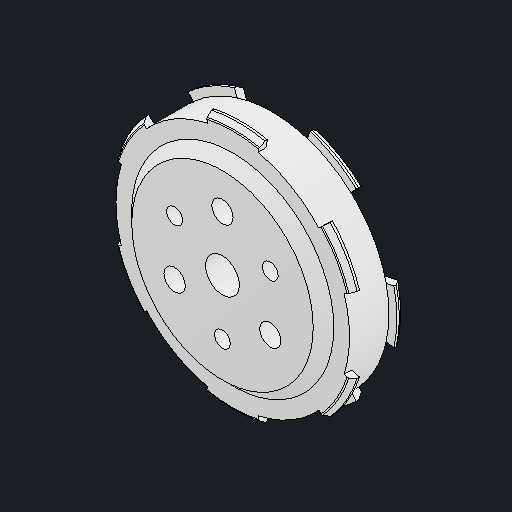
# Autodesk Inventor part: 36mm tamiya-slim-tire-wheel
Saved by Autodesk Inventor 2023.2 (Build 272271030, 271C)
## iProperties
Created: 2023-10-14
Part Number: 36mm tamiya-slim-tire-wheel
Material: Stainless Steel
Document SubType Name: Modeling
Designer: takag
Density: 8 g/cm^3
Appearance: 滑らか - 白
Author: takag
Autodesk Inventor part; units mm, degrees
ref_plane "YZ Plane" through (0, 0, 0) normal (1, 0, 0) x (0, 1, 0)
ref_plane "XZ Plane" through (0, 0, 0) normal (0, 1, 0) x (-1, 0, 0)
ref_plane "XY Plane" through (0, 0, 0) normal (0, 0, 1) x (1, 0, 0)
sketch "スケッチ1" plane through (0, 0, 0) normal (0, 0, 1) x (1, 0, 0)
  circle A0 centre (0, 0) radius 15.8
  dimension "d0" = 31.6
  constraints: 1 centre point, 1 coincident
  measures "d0" diameter of A0
extrude "押し出し1" add sketch "スケッチ1" along normal blind 7.3
sketch "スケッチ2" plane through (0, 0, 7.3) normal (0, 0, 1) x (1, 0, 0)
  circle A0 centre (0, 0) radius 12.8
  circle A1 centre (0, 0) radius 15.8 projected
  dimension "d3" = 3
  constraints: 1 centre point, 1 coincident
  measures "d3" radial gap between concentric circles of A1 A0
extrude "押し出し2" cut sketch "スケッチ2" against normal blind 1.3
sketch "スケッチ3" plane through (0, 0, 7.3) normal (0, 0, 1) x (1, 0, 0)
  circle A0 centre (0, 0) radius 13
  dimension "d6" = 26
  constraints: 1 centre point, 1 coincident
  measures "d6" diameter of A0
ref_plane "Work Plane2" through (0, 0, 7.3) normal (0, 0, 1) x (1, 0, 0)
sketch "スケッチ6" plane through (0, 0, 0) normal (1, 0, 0) x (0, 1, 0)
  line L0 (15.8, 0) -> (15.8, 6) projected
  line L1 (-15.8, 6) -> (15.8, 6) projected
  line L2 (15.8, 5) -> (14.8, 5)
  line L3 (14.8, 5) -> (14.8, 1)
  line L4 (14.8, 1) -> (15.8, 1)
  line L5 (15.8, 1) -> (15.8, 5)
  line L6 (15.8, 0) -> (15.8, 6) projected
  line L7 (12.3846, 7.3) -> (-2.7694, 7.3) projected
  line L8 (0, 7.3) -> (0, 0)
  line L9 (15.8, 0) -> (-15.8, 0) projected
  point P0 (15.8, 1)
  point P1 (15.8, 1)
  dimension "d18" = 1
  dimension "d19" = 1
  dimension "d20" = 1
  constraints: 10 end point, 3 point on line, 2 parallel, 2 perpendicular, 1 horizontal
  measures "d18" distance from line of L1 L2.start
  measures "d19" distance of L0.start point (15.8, 1)
  measures "d20" distance between parallel lines of L0 L3
revolve "回転2" cut sketch "スケッチ6" angle 360 about axis through (0, 0, 7.3) along (0, 0, -1) contours L4 L3 L2 L0
chamfer "面取り1" distance 0.7 distance2 0.5 1 edges at (-15.8, 0, 6) measured on face at (-15.8, 0, 5.5)
chamfer "面取り2" distance 0.7 distance2 0.5 1 edges at (-15.8, 0, 0) measured on face at (-15.8, 0, 0.5)
sketch "スケッチ7" plane through (0, 0, 6) normal (0, 0, 1) x (1, 0, 0)
  line L0 (0, 0) -> (-7.9, 13.6832)
  arc A0 (15.8, 0) -> (15.8, 0) centre (0, 0) ccw projected
  line L1 (-7.9, 13.6832) -> (-3.5699, 16.1832)
  line L2 (-7.9, 13.6832) -> (-12.2301, 11.1832)
  line L3 (-7.9, 13.6832) -> (-2.9, 13.6832) construction
  line L4 (-12.2301, 11.1832) -> (0, 0)
  line L5 (0, 0) -> (-3.5699, 16.1832)
  arc A1 (15.3, 0) -> (15.3, 0) centre (0, 0) ccw projected
  arc A2 (0, 14.8) -> (0, 14.8) centre (0, 0) ccw projected
  line L6 (0, 0) -> (0, 30.7914)
  circle A3 centre (0, 0) radius 14.8 projected
  point P0 (-4.767, 15.0637)
  point P1 (-4.4653, 14.1103)
  point P2 (4.4653, 14.1103)
  point P3 (4.767, 15.0637)
  point P4 (-10.9222, 9.9873)
  point P5 (-3.1881, 14.4525)
  dimension "d28" = 5
  dimension "d29" = 5
  dimension "d30" = 150
  dimension "d94" = 30
  constraints: 14 end point, 2 tangent, 1 equal length, 1 horizontal, 1 point on circle, 1 vertical
  measures "d28" distance of L0.end L1.end
  measures "d29" distance of L0.end L2.end
  measures "d30" angle of L2 L3
  measures "d94" angle of L0 L6
extrude "押し出し4" cut sketch "スケッチ7" against normal blind 1.3 contours A2 L4 A1 L0 | L0 A1 L5 A2 | A1 L4 A0 L0 | L0 A0 L5 A1 | L1 L5 A0 | A0 L4 L2
sketch "スケッチ8" plane through (0, 0, 0) normal (0, 0, -1) x (-1, 0, 0)
  line L0 (0, 0) -> (0, -15.8)
  arc A0 (0, 15.8) -> (0, 15.8) centre (0, 0) ccw projected
  line L1 (0, -15.8) -> (-5, -15.8)
  line L2 (0, -15.8) -> (5, -15.8)
  line L3 (5, -15.8) -> (0, 0)
  line L4 (0, 0) -> (-5, -15.8)
  circle A1 centre (0, 0) radius 14.8 projected
  point P0 (-4.4653, -14.1103)
  point P1 (-4.767, -15.0637)
  point P2 (4.767, -15.0637)
  point P3 (4.4653, -14.1103)
  dimension "d36" = 5
  dimension "d37" = 5
  constraints: 10 end point, 1 perpendicular, 1 point on circle, 1 point on line, 1 vertical
  measures "d36" distance of L0.end L1.end
  measures "d37" distance of L0.end L2.end
extrude "押し出し5" cut sketch "スケッチ8" against normal up to surface (1 mm away) contours L3 A1 L0 | L0 A1 L4 | A1 L3 A0 L0 | L0 A0 L4 A1 | L1 L4 A0 | A0 L3 L2
pattern_circular "Circular Pattern6" count 6 over 360 about axis through (0, 0, 3) along (0, 0, 1) of "押し出し5", "押し出し4"
sketch "スケッチ9" plane through (0, 0, 0) normal (0, 0, -1) x (-1, 0, 0)
  circle A0 centre (0, 0) radius 12.8
  dimension "d93" = 25.6
  constraints: 1 centre point, 1 coincident
  measures "d93" diameter of A0
extrude "押し出し6" cut sketch "スケッチ9" against normal blind 4.5
sketch "スケッチ10" plane through (0, 0, 4.5) normal (0, 0, -1) x (-1, 0, 0)
  circle A0 centre (0, 0) radius 13
  constraints: 1 centre point, 1 coincident
extrude "押し出し7" cut sketch "スケッチ10" against normal blind 1.3
sketch "スケッチ13" plane through (0, 0, 5.8) normal (0, 0, -1) x (-1, 0, 0)
  circle A0 centre (0, 0) radius 3.5
  circle A1 centre (0, 7) radius 2.5
  circle A2 centre (-6.0622, -3.5) radius 2.5
  circle A3 centre (6.0622, -3.5) radius 2.5
  dimension "d53" = 7
  dimension "d54" = 5
  dimension "d55" = 7
  dimension "d58" = 360
  constraints: 4 centre point, 1 coincident, 7 other
  measures "d53" diameter of A0
  measures "d54" diameter of A1
  measures "d55" distance of point (0, 0) A1.centre
extrude "押し出し9" add sketch "スケッチ13" along normal blind 5.8 contours A1 | A2 | A3
sketch "スケッチ14" plane through (0, 0, 5.8) normal (0, 0, -1) x (-1, 0, 0)
  circle A0 centre (0, 0) radius 3.5
  dimension "d62" = 7
  constraints: 1 centre point, 1 coincident
  measures "d62" diameter of A0
extrude "押し出し10" add sketch "スケッチ14" along normal blind 7
sketch "スケッチ15" plane through (0, 7, 0) normal (0, 0, -1) x (-1, 0, 0)
  circle A0 centre (0, 0) radius 2.5 projected
  circle A1 centre (0, 0) radius 1.35
  circle A2 centre (6.0622, -10.5) radius 2.5 projected
  circle A3 centre (-6.0622, -10.5) radius 2.5 projected
  circle A4 centre (6.0622, -10.5) radius 1.35
  circle A5 centre (-6.0622, -10.5) radius 1.35
  point P0 (0, -7)
  dimension "d65" = 2.7
  constraints: 3 centre point, 3 coincident, 2 equal radius
  measures "d65" diameter of A1
extrude "押し出し11" cut sketch "スケッチ15" against normal through all contours A1 | A4 | A5
sketch "スケッチ16" plane through (0, 0, -1.2) normal (0, 0, -1) x (-1, 0, 0)
  circle A0 centre (0, 0) radius 2.15
  dimension "d71" = 4.3
  constraints: 1 centre point, 1 coincident
  measures "d71" diameter of A0
extrude "押し出し12" cut sketch "スケッチ16" against normal through all
sketch "スケッチ17" plane through (0, 0, 7.3) normal (0, 0, 1) x (1, 0, 0)
  circle A0 centre (0, 0) radius 2.15 projected
  circle A1 centre (0, -7) radius 1
  dimension "d74" = 7
  dimension "d75" = 2
  constraints: 1 centre point, 1 coincident
  measures "d74" distance of A0.centre point (0, -7)
  measures "d75" diameter of A1
extrude "押し出し13" cut sketch "スケッチ17" against normal through all contours A1
pattern_circular "円形状パターン5" count 3 over 360 about axis through (0, 0, -1.2) along (0, 0, 1) of "押し出し13"
sketch "スケッチ18" plane through (0, 0, -1.2) normal (0, 0, -1) x (-1, 0, 0)
  circle A0 centre (0, 0) radius 3.5 projected
  point P0 (-3.5, 0)
  constraints: 1 horizontal alignment, 1 other
ref_plane "作業平面1" through (3.5, 0, -1.2) normal (1, 0, 0) x (0, 1, 0)
sketch "スケッチ19" plane through (3.5, 0, -1.2) normal (1, 0, 0) x (0, 1, 0)
  line L0 (2.15, 0) -> (-2.15, 0) projected
  line L1 (0, 0) -> (1, 0)
  line L2 (0, 0) -> (-1, 0)
  line L3 (1, 0) -> (-1, 0)
  line L4 (-1, 0) -> (-1, 3)
  line L5 (-1, 3) -> (1, 3)
  line L6 (1, 3) -> (1, 0)
  circle A0 centre (0, 2) radius 1
  point P0 (0, 1.2)
  point P1 (0, 3)
  point P2 (-1, 2)
  point P3 (1, 2)
  dimension "d81" = 1
  dimension "d82" = 1
  dimension "d83" = 3
  constraints: 12 end point, 2 midpoint, 2 parallel, 2 point on line, 1 collinear, 1 perpendicular, 1 vertical, 3 other
  measures "d81" distance of L1.start L1.end
  measures "d82" distance of L1.start L2.end
  measures "d83" distance of L2.end L4.end
extrude "押し出し14" cut sketch "スケッチ19" against normal blind 7 contours L0 L4 A0 L6 | A0
fillet "フィレット1" radius 0.2 6 edges at (-13.2502, -7.65, 6) (13.2502, 7.65, 6) (-13.2502, 7.65, 6) (13.2502, -7.65, 6) (0, -15.3, 6) (0, 15.3, 6)
fillet "フィレット3" radius 0.2 8 edges at (15.3, 0, 0) (7.65, 13.2502, 0) (-7.65, -13.2502, 0) (-7.65, 13.2502, 0) (-15.3, 0, 0) (7.65, -13.2502, 0) (4.239, -13.3953, 0) (-4.239, -13.3953, 0)
chamfer "Chamfer3" distance 1.3 angle 45 1 edges at (-12.8, 0, 7.3)
sketch "Sketch20" plane through (0, 0, 0) normal (1, 0, 0) x (0, 1, 0)
  line L0 (3.5, 5.8) -> (3.5, -1.2) projected
  line L1 (12.8, 1) -> (12.8, 4.5) projected
  line L2 (3.5, 5.8) -> (-3.5, 5.8) projected
  line L3 (3.5, 5.8) -> (12.8, 5.8)
  line L4 (12.8, 5.8) -> (12.8, 4.5)
  line L5 (12.8, 4.5) -> (3.5, 4.5)
  line L6 (3.5, 4.5) -> (3.5, 5.8)
  line L7 (9.5, 5.8) -> (9.5, 0) projected
  line L8 (4.5, 5.8) -> (4.5, 0) projected
  line L9 (5.65, 7.3) -> (8.35, 7.3) projected
  line L10 (8.35, 0) -> (5.65, 0) projected
  line L11 (5.65, 0) -> (5.65, 7.3) projected
  line L12 (8.35, 0) -> (8.35, 7.3) projected
  point P0 (0, 0)
  point P1 (9.5, 4.5)
  point P2 (4.5, 4.5)
  point P3 (3.5, 4.5)
  point P4 (8.35, 5.8)
  point P5 (8.35, 4.5)
  point P6 (5.65, 4.5)
  point P7 (5.65, 5.8)
  dimension "d101" = 1.3
  constraints: 8 end point, 2 parallel, 1 horizontal, 1 perpendicular, 1 point on line
  measures "d101" distance of L3.end L4.end
extrude "Extrusion15" add sketch "Sketch20" along normal mid plane 0.5 contours L3 L8 L5 L0 | L3 L11 L5 L8 | L3 L7 L5 L12 | L3 L4 L5 L7
pattern_circular "Circular Pattern7" count 3 over 360 about axis through (0, 0, 5.8) along (0, 0, -1) of "Extrusion15"
